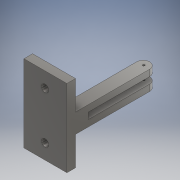
# Autodesk Inventor part: Podstawka
Saved by Autodesk Inventor 2017 (Build 210142000, 142)
## iProperties
Created: 2018-05-29
Part Number: Podstawka
Material: Stainless Steel, Austenitic
Document SubType Name: Modeling
Designer: Pies
Density: 8 g/cm^3
Appearance: Semi-Polished
Author: Pies
Autodesk Inventor part; units mm, degrees
ref_plane "YZ Plane" through (0, 0, 0) normal (1, 0, 0) x (0, 1, 0)
ref_plane "XZ Plane" through (0, 0, 0) normal (0, 1, 0) x (-1, 0, 0)
ref_plane "XY Plane" through (0, 0, 0) normal (0, 0, 1) x (1, 0, 0)
sketch "Sketch1" plane through (0, 0, 0) normal (0, 0, 1) x (1, 0, 0)
  line L0 (-3, 38.5) -> (-3, 0)
  line L1 (-3, 0) -> (3, 0)
  line L2 (3, 0) -> (3, 38.5)
  line L3 (-3, 38.5) -> (-3, 36)
  arc A0 (3, 38.5) -> (-3, 38.5) centre (0, 38.5) ccw
  point P0 (0, 0)
  constraints: 8 end point, 2 perpendicular, 2 point on circle, 1 centre point, 1 point on line, 1 tangent
extrude "Extrusion1" add sketch "Sketch1" along normal blind 9
sketch "Sketch2" plane through (3, 0, 0) normal (1, 0, 0) x (0, 0, -1)
  line L0 (-3, 41.5) -> (-6, 41.5)
  line L1 (-6, 41.5) -> (-6, 10)
  line L2 (-6, 10) -> (-3, 10)
  line L3 (-3, 10) -> (-3, 41.5)
  point P0 (0, 0)
  point P1 (-9, 41.5)
  constraints: 8 end point, 2 perpendicular, 1 vertical
extrude "Extrusion2" cut sketch "Sketch2" against normal through all
sketch "Sketch3" plane through (0, 0, 9) normal (0, 0, 1) x (1, 0, 0)
  line L0 (-3, 38.5) -> (-3, 0) projected
  line L1 (-3, 4) -> (3, 4)
  line L2 (3, 0) -> (-17, 0)
  line L3 (-17, 0) -> (-17, 4)
  line L4 (-17, 4) -> (3, 4)
  line L5 (3, 0) -> (3, 4)
  line L6 (3, 0) -> (3, 38.5) projected
  point P0 (0, 0)
  dimension "d77" = 20
  constraints: 10 end point, 2 perpendicular, 2 point on line, 1 collinear, 1 horizontal, 1 parallel
  measures "d77" distance of L3.end L4.end
sketch "Sketch8" plane through (0, 0, 9) normal (0, 0, 1) x (1, 0, 0)
  arc A0 (3, 38.5) -> (-3, 38.5) centre (0, 38.5) ccw construction
  line L0 (0, 41.5) -> (0, 38.75) construction
  circle A1 centre (0, 38.75) radius 0.5
  point P0 (0, 0)
  dimension "d68" = 2.75
  dimension "d69" = 1
  constraints: 2 end point, 1 centre point, 1 coincident, 1 point on circle, 1 vertical
  measures "d68" distance of L0.start L0.end
  measures "d69" diameter of A1
extrude "Extrusion6" cut sketch "Sketch8" against normal through all
extrude "Extrusion7" add sketch "Sketch3" along normal blind 13.5 and the other way blind 22.5
sketch "Sketch10" plane through (-3, 4, 9) normal (0, 1, 0) x (1, 0, 0)
  point P0 (3, 9)
  point P1 (6, 22.5)
  point P2 (6, -13.5)
  point P3 (-4.142, -6.5)
  point P4 (-4.142, 15.5)
hole "Hole4" at (-7.142, 4, 15.5) at (-7.142, 4, -6.5) direction (0, -1, 0) diameter 3.4 end through all clearance for "Hex Head Cap Screw ISO 24017" size "M3" standard "ISO"
body "Solid1"
